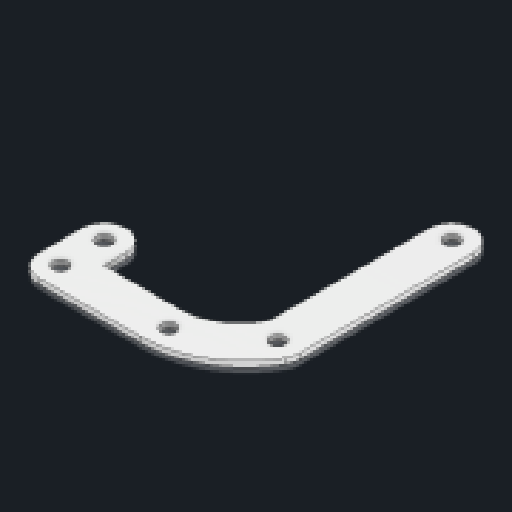
# Autodesk Inventor part: MOGO Funnel
Saved by Autodesk Inventor 2025 (Build 290162000, 162)
## iProperties
Created: 2024-12-27
Part Number: MOGO Funnel
Material: Acetal Resin, White
Document SubType Name: Sheet Metal
Designer: Averey Ku
Density: 1.425 g/cm^3
Appearance: Smooth - White
Flat Pattern Width: 7.62135 cm
Flat Pattern Length: 6.35406 cm
Flat Pattern Area: 48.4265 cm^2
Sheet Metal Rule: Default_mm
Sheet Metal Width: 3.001 in
Sheet Metal Length: 2.502 in
Sheet Metal Area: 7.506 in^2
Mass: 3.54322 g
Surface Area: 36.7606 cm^2
Volume: 2.48647 cm^3
d7: 0.165 in
Author: Averey Ku
Autodesk Inventor part; units mm, degrees
ref_plane "YZ Plane" through (0, 0, 0) normal (1, 0, 0) x (0, 1, 0)
ref_plane "XZ Plane" through (0, 0, 0) normal (0, 1, 0) x (-1, 0, 0)
ref_plane "XY Plane" through (0, 0, 0) normal (0, 0, 1) x (1, 0, 0)
sketch "main" plane through (0, 0, 0) normal (0, 0, 1) x (1, 0, 0)
  circle A0 centre (10.4433, 33.6894) radius 2.1844
  circle A1 centre (19.1546, 24.4481) radius 2.1844
  arc A2 (14.5223, 20.0458) -> (23.795, 28.8419) centre (19.1546, 24.4481) ccw
  line L0 (14.9701, 38.1619) -> (23.795, 28.8419)
  circle A3 centre (-17.8109, -10.3972) radius 2.1844
  circle A4 centre (17.0343, -47.3627) radius 2.1844
  arc A5 (21.39, -51.9834) -> (21.655, -43.007) centre (17.0343, -47.3627) ccw
  arc A6 (15.156, 37.9656) -> (6.0681, 38.3102) centre (10.4433, 33.6894) ccw
  line L1 (6.0681, 38.3102) -> (-15.262, 18.1133)
  line L2 (-10.4267, -8.9732) -> (21.655, -43.007)
  line L3 (14.5223, 20.0458) -> (10.1592, 24.6941)
  line L4 (1.4674, 33.9539) -> (1.4319, 33.9917)
  line L5 (-5.9349, 9.455) -> (10.1592, 24.6941)
  circle A7 centre (-12.7, 11.9618) radius 2.0955
  arc A8 (-5.9349, 9.455) -> (-10.4267, -8.9732) centre (6.0813, -3.2354) ccw
  arc A9 (-15.262, 18.1133) -> (-23.9645, -11.9645) centre (5.9931, -4.3343) ccw
  arc A10 (12.4136, -51.7183) -> (21.655, -43.007) centre (17.0343, -47.3627) ccw
  arc A11 (-23.9645, -11.9645) -> (-22.4316, -14.7529) centre (-17.8109, -10.3972) ccw
  line L6 (12.4136, -51.7183) -> (-22.4316, -14.7529)
  point P0 (-4.8343, 8.0815)
  dimension "d7" = 4.191
  measures "d7" diameter of A7
sketch "Sketch1" plane through (0, 0, 0) normal (0, 1, 0) x (-1, 0, 0)
  circle A0 centre (0, 12.7) radius 2.1844
  circle A1 centre (0, 0) radius 2.1844
  arc A2 (-6.3904, -0.0259) -> (6.3905, 0.0143) centre (0, 0) ccw
  line L0 (6.3618, 12.8494) -> (6.3905, 0.0143)
  circle A3 centre (-50.8, 0) radius 2.1844
  circle A4 centre (-50.8, -50.8) radius 2.1844
  arc A5 (-50.8, -57.15) -> (-44.45, -50.8) centre (-50.8, -50.8) ccw
  arc A6 (6.3624, 12.5791) -> (-0.0142, 19.0635) centre (0, 12.7) ccw
  line L1 (-0.0142, 19.0635) -> (-29.3891, 18.9978)
  line L2 (-44.45, -4.0289) -> (-44.45, -50.8)
  line L3 (-6.3904, -0.0259) -> (-6.377, 6.3492)
  line L4 (-6.3501, 19.0493) -> (-6.35, 19.1012)
  line L5 (-28.5411, 6.2997) -> (-6.377, 6.3492)
  circle A7 centre (-31.7443, 12.7641) radius 2.0955
  arc A8 (-28.5411, 6.2997) -> (-44.45, -4.0289) centre (-28.502, -11.177) ccw
  arc A9 (-29.3891, 18.9978) -> (-56.3528, 3.0805) centre (-29.3199, -11.9162) ccw
  arc A10 (-57.15, -50.8) -> (-44.45, -50.8) centre (-50.8, -50.8) ccw
  arc A11 (-56.3528, 3.0805) -> (-57.1501, 0) centre (-50.8, 0) ccw
  line L6 (-57.15, -50.8) -> (-57.1501, 0)
  point P0 (0, 0)
  point P1 (-50.8, -57.15)
  constraints: 1 other
extrude "Extrusion1" add sketch "Sketch1" along normal blind 1.5875
equation "\"BendRadius\" = Thickness"
equation "\"BendReliefWidth\" = Thickness"
equation "\"BendReliefDepth\" = 0.5 * Thickness"
equation "\"CornerReliefSize\" = 4 * Thickness"
equation "\"MinimumRemnant\" = 2 * Thickness"
equation "\"TransitionRadius\" = BendRadius"
equation "\"JacobiRadiusSize\" = BendRadius"
equation "\"GapSize\" = Thickness"
equation "\"Thickness\" = 1.5875"
body "Solid1"
